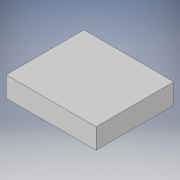
# Autodesk Inventor part: MP#
Saved by Autodesk Inventor 2017 (Build 210142000, 142)
## iProperties
Created: 2019-05-26
Part Number: MP#
Material: Generic
Document SubType Name: Modeling
Designer: Mitch
Density: 1 g/cm^3
Appearance: Default
Author: Mitch
Autodesk Inventor part; units mm, degrees
ref_plane "YZ Plane" through (0, 0, 0) normal (1, 0, 0) x (0, 1, 0)
ref_plane "XZ Plane" through (0, 0, 0) normal (0, 1, 0) x (-1, 0, 0)
ref_plane "XY Plane" through (0, 0, 0) normal (0, 0, 1) x (1, 0, 0)
sketch "Sketch1" plane through (0, 0, 0) normal (0, 1, 0) x (-1, 0, 0)
  line L0 (0, 0) -> (20.5232, 0)
  line L1 (20.5232, 0) -> (20.5232, -17.78)
  line L2 (20.5232, -17.78) -> (0, -17.78)
  line L3 (0, -17.78) -> (0, 0)
  dimension "d0" = 20.5232
  dimension "d1" = 17.78
  constraints: 8 end point, 2 parallel, 1 horizontal, 1 perpendicular
  measures "d0" distance of L1.end L2.end
  measures "d1" distance of L0.end L1.end
extrude "Extrusion1" add sketch "Sketch1" along normal blind 4.6228
body "Solid1"
